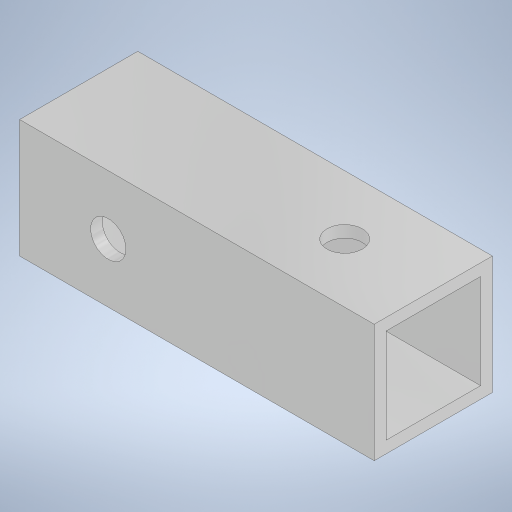
# Autodesk Inventor part: omu_k_jo_5
Saved by Autodesk Inventor 2024.2 (Build 282272000, 272)
## iProperties
Created: 2024-01-23
Part Number: omu_k_jo_5
Material: アルミニウム 6061-AHC
Document SubType Name: Modeling
Designer: fhbdh
Density: 2.7 g/cm^3
Appearance: アルミニウム - ダーク
Author: fhbdh
Autodesk Inventor part; units mm, degrees
ref_plane "YZ Plane" through (0, 0, 0) normal (1, 0, 0) x (0, 1, 0)
ref_plane "XZ Plane" through (0, 0, 0) normal (0, 1, 0) x (-1, 0, 0)
ref_plane "XY Plane" through (0, 0, 0) normal (0, 0, 1) x (1, 0, 0)
sketch "スケッチ1" plane through (0, 0, 0) normal (1, 0, 0) x (0, 1, 0)
  line L0 (-5, -5) -> (5, -5)
  line L1 (5, -5) -> (5, 5)
  line L2 (5, 5) -> (-5, 5)
  line L3 (-5, 5) -> (-5, -5)
  line L4 (-5, -5) -> (5, 5) construction
  line L5 (5, -5) -> (-5, 5) construction
  line L6 (4, 4) -> (4, -4)
  line L7 (4, -4) -> (-4, -4)
  line L8 (-4, -4) -> (-4, 4)
  line L9 (-4, 4) -> (4, 4)
  point P0 (0, 0)
  dimension "d0" = 1
  dimension "d1" = 10
  dimension "d2" = 10
  constraints: 20 end point, 4 parallel, 2 midpoint, 2 perpendicular, 1 horizontal, 3 other
  measures "d0" distance between parallel lines of L1 L6
  measures "d1" distance of L0.end L1.end
  measures "d2" distance of L1.end L2.end
extrude "押し出し1" add sketch "スケッチ1" along normal blind 30
sketch "スケッチ2" plane through (0, -5, 5) normal (0, 0, 1) x (1, 0, 0)
  line L0 (0, 5) -> (30, 5) construction
  line L1 (30, 9) -> (30, 1) projected
  circle A0 centre (7.5, 5) radius 1.5
  line L2 (0, 10) -> (0, 0) projected
  dimension "d5" = 3
  dimension "d6" = 7.5
  constraints: 2 end point, 1 centre point, 1 midpoint, 1 point on line
  measures "d5" diameter of A0
  measures "d6" distance from line of L2 A0.centre
extrude "押し出し2" cut sketch "スケッチ2" against normal through all
sketch "スケッチ3" plane through (0, 5, 5) normal (0, 1, 0) x (1, 0, 0)
  line L0 (0, 5) -> (30, 5) construction
  line L1 (30, 0) -> (30, 10) projected
  circle A0 centre (22.5, 5) radius 1.5
  dimension "d9" = 3
  dimension "d10" = 7.5
  constraints: 2 end point, 1 centre point, 1 midpoint, 1 point on line
  measures "d9" diameter of A0
  measures "d10" distance from line of L1 A0.centre
extrude "押し出し3" cut sketch "スケッチ3" against normal through all
sketch "スケッチ4" plane through (0, 5, 5) normal (0, 1, 0) x (1, 0, 0)
  line L0 (30, 10) -> (30, 0) projected
  line L1 (0, 10) -> (0, 0) projected
  circle A0 centre (22.5, 5) radius 1.5 projected
  point P0 (0, 5)
  dimension "d13" = 30
  dimension "d14" = 22.5
  measures "d13" distance between parallel lines of L0 L1
  measures "d14" distance from line of A0.centre L1
sketch "スケッチ5" plane through (0, -5, 5) normal (0, 0, 1) x (1, 0, 0)
  line L0 (30, 10) -> (30, 0) projected
  line L1 (0, 10) -> (0, 0) projected
  circle A0 centre (7.5, 5) radius 1.5 projected
  point P0 (0, 5)
  dimension "d16" = 7.5
  measures "d16" distance from line of A0.centre L1
